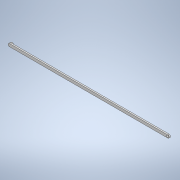
# Autodesk Inventor part: eslasbon_2
Saved by Autodesk Inventor 2021 (Build 250183000, 183)
## iProperties
Created: 2021-07-12
Part Number: eslasbon_2
Material: Genérico
Document SubType Name: Modeling
Designer: Leonardo Fabio Mercado Benítez
Density: 1 g/cm^3
Appearance: Valor por defecto
Author: Leonardo Fabio Mercado Benítez
Autodesk Inventor part; units mm, degrees
ref_plane "YZ Plane" through (0, 0, 0) normal (1, 0, 0) x (0, 1, 0)
ref_plane "XZ Plane" through (0, 0, 0) normal (0, 1, 0) x (-1, 0, 0)
ref_plane "XY Plane" through (0, 0, 0) normal (0, 0, 1) x (1, 0, 0)
sketch "Boceto1" plane through (0, 0, 0) normal (0, 0, 1) x (1, 0, 0)
  arc A0 (0, 3.175) -> (0, -3.175) centre (0, 0) ccw
  line L0 (360.825, 0) -> (364, 0)
  arc A1 (364, -3.175) -> (364, 3.175) centre (364, 0) ccw
  line L1 (0, 3.175) -> (364, 3.175)
  line L2 (364, -3.175) -> (0, -3.175)
  dimension "d0" = 6.35
  dimension "d1" = 364
  dimension "d2" = 6.35
  constraints: 6 end point, 4 point on circle, 2 centre point, 2 coincident, 2 tangent, 1 horizontal
  measures "d0" diameter of A0
  measures "d1" distance of A0.centre L0.end
  measures "d2" diameter of A1
extrude "Extrusión1" add sketch "Boceto1" along normal blind 3.175
sketch "Boceto2" plane through (0, 0, 0) normal (0, 0, -1) x (-1, 0, 0)
  circle A0 centre (0, 0) radius 2.675
  dimension "d5" = 5.35
  constraints: 1 centre point, 1 coincident
  measures "d5" diameter of A0
extrude "Extrusión2" add sketch "Boceto2" along normal blind 3.175
sketch "Boceto3" plane through (0, 0, 0) normal (0, 0, -1) x (-1, 0, 0)
  arc A0 (-364, 3.175) -> (-364, -3.175) centre (-364, 0) ccw projected
  circle A1 centre (-364, 0) radius 2.675
  point P0 (0, 0)
  dimension "d8" = 5.35
  constraints: 1 centre point, 1 coincident
  measures "d8" diameter of A1
extrude "Extrusión3" cut sketch "Boceto3" against normal blind 3.175
